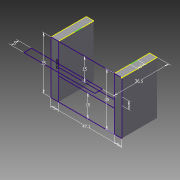
# Autodesk Inventor part: 100x0y0z_0x0y0z
Saved by Autodesk Inventor 2015 (Build 190159000, 159)
## iProperties
Created: 2016-12-15
Part Number: 100x0y0z_0x0y0z
Material: Generic
Document SubType Name: Modeling
Designer: Rudge-Top
Density: 1 g/cm^3
Appearance: Default
Author: Rudge-Top
Autodesk Inventor part; units mm, degrees
ref_plane "YZ Plane" through (0, 0, 0) normal (1, 0, 0) x (0, 1, 0)
ref_plane "XZ Plane" through (0, 0, 0) normal (0, 1, 0) x (-1, 0, 0)
ref_plane "XY Plane" through (0, 0, 0) normal (0, 0, 1) x (1, 0, 0)
sketch "Sketch1" plane through (0, 0, 0) normal (0, 1, 0) x (-1, 0, 0)
  line L0 (0, 0) -> (47.1, 0)
  line L1 (47.1, 0) -> (47.1, -35)
  line L2 (47.1, -35) -> (0, -35)
  line L3 (0, -35) -> (0, 0)
  line L4 (47.1, 0) -> (42.1, 0)
  line L5 (42.1, 0) -> (42.1, -35)
  line L6 (42.1, -35) -> (47.1, -35)
  line L7 (47.1, -35) -> (47.1, 0)
  line L8 (42.1, -15) -> (5, -15)
  line L9 (0, -11) -> (0, -16)
  line L10 (5, -20) -> (42.1, -20)
  line L11 (42.1, -20) -> (42.1, -15)
  line L12 (0, 0) -> (5, 0)
  line L13 (5, 0) -> (5, -35)
  line L14 (5, -35) -> (0, -35)
  line L15 (0, -35) -> (0, 0)
  dimension "d0" = 47.1
  dimension "d1" = 35
  dimension "d2" = 5
  dimension "d3" = 5
  dimension "d4" = 15
  dimension "d6" = 5
  dimension "d7" = 35
  dimension "d15" = 15
  constraints: 32 end point, 8 parallel, 5 point on line, 4 horizontal, 4 perpendicular
  measures "d0" distance of L1.end L2.end
  measures "d1" distance of L0.end L1.end
  measures "d2" distance of L6.end L5.end
  measures "d3" distance of L9.end L9.start
  measures "d4" distance between parallel lines of L0 L8
  measures "d6" distance of L13.end L14.end
  measures "d7" distance of L12.end L13.end
  measures "d15" distance between parallel lines of L2 L10
extrude "Extrusion1" add sketch "Sketch1" along normal blind 23.5 contours L0 L13 L2 L3 | L0 L1 L2 L5
sketch "Sketch2" plane through (-47.1, 0, 0) normal (0, 0, 1) x (1, 0, 0)
  line L0 (0, 0) -> (5, 0) projected
  line L1 (5, 0) -> (5, 23.5) projected
  line L2 (0, 23.5) -> (5, 23.5) projected
  line L3 (0, 0) -> (0, 23.5) projected
  line L4 (42.1, 0) -> (47.1, 0) projected
  line L5 (47.1, 0) -> (47.1, 23.5) projected
  line L6 (42.1, 23.5) -> (47.1, 23.5) projected
  line L7 (42.1, 0) -> (42.1, 23.5) projected
  line L8 (5, 0) -> (5, 23.5) projected
  line L9 (42.1, 0) -> (42.1, 23.5) projected
  line L10 (42.1, 15.5) -> (42.1, 10.5)
  line L11 (5, 10.5) -> (5, 15.5)
  line L12 (47.1, 0) -> (47.1, 23.5) projected
  line L13 (0, 0) -> (0, 23.5) projected
  line L14 (47.1, -13) -> (0, -13)
  line L15 (0, -13) -> (0, -18)
  line L16 (0, -18) -> (47.1, -18)
  line L17 (47.1, -18) -> (47.1, -13)
  dimension "d10" = 5
  dimension "d16" = 5
  dimension "d17" = 36.5
  constraints: 12 end point, 4 point on line, 3 parallel, 1 horizontal, 1 perpendicular
  measures "d10" distance of L10.start L10.end
  measures "d16" distance of L15.end L14.end
  measures "d17" distance between parallel lines of L6 L14
sketch "Sketch3" plane through (0, 0, 0) normal (0, -1, 0) x (1, 0, 0)
  line L0 (-43.6752, -16.6981) -> (-43.6752, -10.5412) construction
  line L1 (-43.6752, -10.5412) -> (-38.9883, -10.5412) construction
  line L2 (-38.9883, -10.5412) -> (-38.9883, -16.6981) construction
  line L3 (-38.9883, -16.6981) -> (-43.6752, -16.6981) construction
  point P0 (0, 0)
  constraints: 2 other
body "Solid1"
